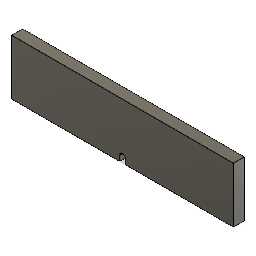
Table_17p1_Problem_3 (Autodesk Fusion 360 design; units mm, degrees)
Autodesk Fusion 360 part; units mm, degrees
sketch "Sketch1" plane through (0, 0, 0) normal (0, 0, 1) x (1, 0, 0)
  line L0 (-100, 0) -> (-100, 25)
  line L1 (-100, 25) -> (100, 25)
  line L2 (100, 25) -> (100, 0)
  line L3 (100, 0) -> (100, -25)
  line L4 (100, -25) -> (2.5, -25)
  line L5 (2.5, -25) -> (2.5, -20)
  arc A0 (2.5, -20) -> (-2.5, -20) centre (0, -20) ccw
  line L6 (-2.5, -20) -> (-2.5, -25)
  line L7 (-2.5, -25) -> (-100, -25)
  line L8 (-100, -25) -> (-100, 0)
  line L9 (-100, 0) -> (100, 0) construction
  line L10 (0, 0) -> (0, -20) construction
  line L11 (-100, -17.5) -> (100, -17.5) construction
  dimension "Total_Width" = 200
  dimension "Total_Height" = 50
  dimension "Notch_Radius" = 2.5
  dimension "Notch_Height" = 7.5
  constraint vertical L0
  constraint perpendicular L0 L1
  constraint perpendicular L1 L2
  constraint perpendicular L1 L3
  constraint perpendicular L2 L4
  constraint perpendicular L4 L5
  constraint tangent L5 A0
  constraint tangent A0 L6
  constraint perpendicular L4 L6
  constraint perpendicular L2 L7
  constraint perpendicular L4 L8
  constraint equal L0 L2
  constraint equal L3 L8
  constraint equal L5 L6
  constraint coincident L10.start origin
  constraint coincident A0.centre L10.end
  constraint perpendicular L9 L10
  constraint coincident L10.start L9
  constraint coincident L8 L11.start
  constraint coincident L3 L11.end
  constraint horizontal L11
  constraint tangent A0 L11
  constraint equal L0 L8
  constraint equal L4 L7
  measures "Total_Width" distance of L0.start L2.end
  measures "Total_Height" distance of L1 L7
  measures "Notch_Radius" radius of A0
  measures "Notch_Height" distance of L4 L11
extrude "Extrude1" add sketch "Sketch1" along normal mid plane 10
equation "Thickness = 1 cm"
